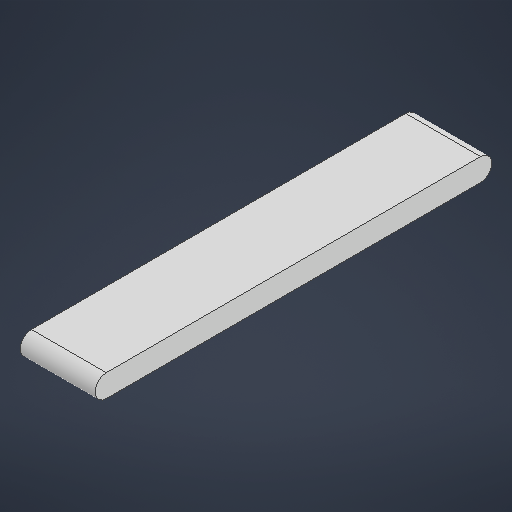
# Autodesk Inventor part: Stainless Steel Mini Conveyor, DC 12 V
Saved by Autodesk Inventor 2027 (Build 310192000, 192)
## iProperties
Created: 2026-04-16
Part Number: Stainless Steel Mini Conveyor, DC 12 V
Material: Generic
Document SubType Name: Modeling
Designer: ratik
Density: 1 g/cm^3
Appearance: Default
Author: ratik
Autodesk Inventor part; units mm, degrees
ref_plane "YZ Plane" through (0, 0, 0) normal (1, 0, 0) x (0, 1, 0)
ref_plane "XZ Plane" through (0, 0, 0) normal (0, 1, 0) x (-1, 0, 0)
ref_plane "XY Plane" through (0, 0, 0) normal (0, 0, 1) x (1, 0, 0)
sketch "Sketch1" plane through (0, 0, 0) normal (1, 0, 0) x (0, 1, 0)
  line L0 (3.2464, 201.4342) -> (3.2464, -298.5658)
  line L1 (33.2464, -298.5658) -> (33.2464, 201.4342)
  arc A0 (33.2464, 201.4342) -> (3.2464, 201.4342) centre (18.2464, 201.4342) ccw
  arc A1 (3.2464, -298.5658) -> (33.2464, -298.5658) centre (18.2464, -298.5658) ccw
  point P0 (0, 0)
  dimension "d0" = 500
  dimension "d1" = 30
  dimension "d2" = 30
  dimension "d3" = 30
  constraints: 4 end point, 4 point on circle, 2 centre point, 1 parallel
  measures "d0" distance of L1.start L1.end
  measures "d1" distance of L0.end L1.start
  measures "d2" diameter of A0
  measures "d3" diameter of A1
extrude "Extrusion1" add sketch "Sketch1" along normal blind 100
body "Solid1"
